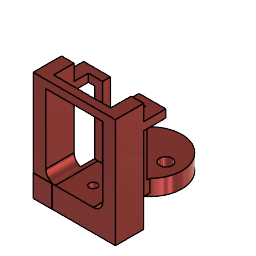
Hexapod Assembly (Autodesk Fusion 360 archive; units mm, degrees)
design "Coxa V1"
part number: 2026-04-28-18-44-43-401
Autodesk Fusion 360 part; units mm, degrees
note: some values were not read from the file. Chosen so that the rebuilt part matches the saved one: which face or edge a step refers to; which pieces of a blend or face edit are solid. Set by a fixed rule: which sketch regions a step uses.
sketch "Sketch1" plane through (0, 0, 0) normal (0, 0, 1) x (1, 0, 0)
sketch "Sketch2" plane through (0, 0, 0) normal (0, 0, 1) x (1, 0, 0)
  circle A0 centre (14.9677, 30.0451) radius 10
  dimension "d1" = 20
  measures "d1" diameter of A0
extrude "Extrude1" add sketch "Sketch2" along normal blind 5
sketch "Sketch3" plane through (0, 0, 5) normal (0, 0, 1) x (-1, 0, 0)
  circle A0 centre (-14.9677, -30.0451) radius 10
  line L0 (-8, -27.0451) -> (-22, -27.0451)
  line L1 (-22, -27.0451) -> (-22, -12.0451)
  line L2 (-22, -12.0451) -> (-8, -12.0451)
  line L3 (-8, -12.0451) -> (-8, -27.0451)
  dimension "d4" = 14
  dimension "d5" = 15
  dimension "d6" = 3
  constraint horizontal L0
  constraint vertical L1
  constraint horizontal L2
  constraint vertical L3
  measures "d4" distance of L0.start L0.end
  measures "d5" distance of L0.start L2.end
  measures "d6" distance of A0.centre L0
extrude "Extrude2" cut sketch "Sketch3" against normal blind 4 contours A0 L0 L1 L3 | A0 L1 L2 L3 picked at (-15.2391, -24.7211)
extrude "Extrude3" add 1 faces at (12.6667, 27.0451, 3.6667) along direction (0, -1, 0) blind 15
sketch "Sketch4" plane through (0, 0, 5) normal (0, 0, 1) x (-1, 0, 0)
extrude "Extrude4" add 1 faces at (12.6667, 12.0451, 3.6667) along direction (0, -1, 0) blind 6
sketch "Sketch5" plane through (8, 0, 0) normal (-1, 0, 0) x (0, -1, 0)
sketch "Sketch6" plane through (0, 0, 5) normal (0, 0, 1) x (1, 0, 0)
sketch "Sketch7" plane through (8, 0, 0) normal (-1, 0, 0) x (0, -1, 0)
sketch "Sketch8" plane through (0, 0, 1) normal (0, 0, -1) x (1, 0, 0)
sketch "Sketch9" plane through (22, 0, 0) normal (1, 0, 0) x (0, 1, 0)
  line L0 (22.9355, 1) -> (22.9355, 5)
  line L1 (22.9355, 5) -> (6.0451, 5)
  line L2 (6.0451, 5) -> (6.0451, 1)
  line L3 (6.0451, 1) -> (22.9355, 1)
  line L4 (15, 1) -> (15, 5)
  constraint coincident L3 L4.start
  constraint coincident L1 L4.end
  constraint perpendicular L1 L4
extrude "Extrude5" add sketch "Sketch9" along normal blind 2.5 contours L1 L2 L3 L4
sketch "Sketch10" plane through (8, 0, 0) normal (-1, 0, 0) x (0, -1, 0)
  line L0 (-15, 1) -> (-6, 1)
  line L1 (-6, 1) -> (-6, 5)
  line L2 (-6, 5) -> (-15, 5)
  line L3 (-15, 5) -> (-15, 1)
  constraint horizontal L0
  constraint vertical L1
  constraint horizontal L2
  constraint vertical L3
extrude "Extrude6" add sketch "Sketch10" along normal blind 2.5
sketch "Sketch11" plane through (8, 0, 0) normal (-1, 0, 0) x (0, -1, 0)
sketch "Sketch12" plane through (0, 0, 5) normal (0, 0, 1) x (-1, 0, 0)
  arc A0 (-22, -22.9355) -> (-8, -22.8721) centre (-14.9677, -30.0451) ccw
  line L0 (-8, -22.8721) -> (-8, -15)
  line L1 (-8, -15) -> (-5.5, -15)
  line L2 (-5.5, -15) -> (-5.5, -6)
  line L3 (-5.5, -6) -> (-8, -6)
  line L4 (-8, -6) -> (-8, -6.0451)
  line L5 (-8, -6.0451) -> (-24.5, -6.0451)
  line L6 (-24.5, -6.0451) -> (-24.5, -15)
  line L7 (-24.5, -15) -> (-22, -15)
  line L8 (-22, -15) -> (-22, -22.9355)
  line L9 (-24.5, -6.0451) -> (-5.5, -6.0451)
  line L10 (-5.5, -6.0451) -> (-5.5, -15)
  line L11 (-5.5, -15) -> (-24.5, -15)
  line L12 (-24.5, -15) -> (-24.5, -6.0451)
  line L13 (-22, -15) -> (-8, -15)
  line L14 (-8, -15) -> (-8, -6)
  line L15 (-8, -6) -> (-22, -6)
  line L16 (-22, -6) -> (-22, -15)
  constraint horizontal L9
  constraint vertical L10
  constraint horizontal L11
  constraint vertical L12
  constraint coincident L1.end L2.start
  constraint coincident L5.end L6.start
  constraint horizontal L13
  constraint vertical L14
  constraint horizontal L15
  constraint vertical L16
  constraint coincident L3.end L4.start
  constraint coincident L7.end L8.start
extrude "Extrude7" add sketch "Sketch12" along normal blind 35 contours L5 L6 L7 L9 L11 L12 L16 | L1 L2 L9 L10 L11 L14
sketch "Sketch13" plane through (0, 0, 40) normal (0, 0, 1) x (-1, 0, 0)
  line L0 (-8, -15) -> (-5.5, -15)
  line L1 (-5.5, -15) -> (-5.5, -6.0451)
  line L2 (-5.5, -6.0451) -> (-8, -6.0451)
  line L3 (-8, -6.0451) -> (-8, -15)
  line L4 (-5.5, -15) -> (-24.5, -15)
  line L5 (-24.5, -15) -> (-24.5, -6)
  line L6 (-24.5, -6) -> (-5.5, -6)
  line L7 (-5.5, -6) -> (-5.5, -15)
  constraint horizontal L4
  constraint vertical L5
  constraint horizontal L6
  constraint vertical L7
  constraint coincident L0.end L1.start
extrude "Extrude8" add sketch "Sketch13" along normal blind 2.5
sketch "Sketch14" plane through (0, 0, 5) normal (0, 0, 1) x (-1, 0, 0)
  circle A0 centre (-10, -30) radius 2
  circle A1 centre (-20, -30) radius 2
  dimension "d21" = 4
  dimension "d22" = 4
  measures "d21" diameter of A0
  measures "d22" diameter of A1
extrude "Extrude9" cut sketch "Sketch14" against normal blind 10
sketch "Sketch15" plane through (0, 0, 5) normal (0, 0, 1) x (-1, 0, 0)
  line L0 (-16.4081, -6.0596) -> (-16.4081, -12.0596)
  line L1 (-24.4681, -12.0596) -> (-5.5251, -12.0596)
  circle A0 centre (-14.9966, -12.0596) radius 1.25
  dimension "d25" = 6
  dimension "d26" = 2.5
  constraint vertical L0
  constraint horizontal L1
  constraint midpoint L1 A0.centre
  measures "d25" distance of L0.start L0.end
  measures "d26" diameter of A0
extrude "Extrude10" cut sketch "Sketch15" against normal blind 10
sketch "Sketch16" plane through (0, 0, 40) normal (0, 0, -1) x (1, 0, 0)
sketch "Sketch17" plane through (0, 0, 42.5) normal (0, 0, 1) x (-1, 0, 0)
  line L0 (-5.5, -6) -> (-24.5, -6)
  line L1 (-24.5, -6) -> (-24.5, -15)
  line L2 (-24.5, -15) -> (-5.5, -15)
  line L3 (-5.5, -15) -> (-5.5, -6)
sketch "Sketch18" plane through (0, 6.0451, 0) normal (0, -1, 0) x (1, 0, 0)
sketch "Sketch19" plane through (0, 0, 1) normal (0, 0, -1) x (1, 0, 0)
sketch "Sketch20" plane through (0, 0, 1) normal (0, 0, -1) x (1, 0, 0)
  circle A0 centre (14.9966, -12.0596) radius 1.25
  arc A1 (22, -22.9355) -> (8, -22.8721) centre (14.9677, -30.0451) ccw
  line L0 (22, -22.9355) -> (22, -15)
  line L1 (22, -15) -> (24.5, -15)
  line L2 (24.5, -15) -> (24.5, -6.0451)
  line L3 (24.5, -6.0451) -> (8, -6.0451)
  line L4 (8, -6.0451) -> (8, -6)
  line L5 (8, -6) -> (5.5, -6)
  line L6 (5.5, -6) -> (5.5, -15)
  line L7 (5.5, -15) -> (8, -15)
  line L8 (8, -15) -> (8, -22.8721)
  line L9 (24.5, -15) -> (5.5, -15)
  line L10 (5.5, -15) -> (5.5, -6)
  line L11 (5.5, -6) -> (24.5, -6)
  line L12 (24.5, -6) -> (24.5, -15)
  constraint horizontal L9
  constraint vertical L10
  constraint horizontal L11
  constraint vertical L12
  constraint coincident L5.end L6.start
  constraint coincident L1.end L2.start
extrude "Extrude11" add sketch "Sketch20" along normal blind 3 contours L1 L2 L3 L4 L5 L6 L7 L9 L10 L11 L12
sketch "Sketch21" plane through (0, 0, 0) normal (0, 0, -1) x (1, 0, 0)
  circle A0 centre (10, -30) radius 2
sketch "Sketch22" plane through (0, 0, 42.5) normal (0, 0, 1) x (-1, 0, 0)
sketch "Sketch23" plane through (0, 0, 0) normal (0, 1, 0) x (1, 0, 0)
sketch "Sketch24" plane through (0, 15, 0) normal (0, 1, 0) x (-1, 0, 0)
sketch "Sketch25" plane through (0, 0, 5) normal (0, 0, 1) x (-1, 0, 0)
sketch "Sketch26" plane through (0, 0, 5) normal (0, 0, 1) x (-1, 0, 0)
  line L0 (-8, -22) -> (-10.5, -22)
  line L1 (-10.5, -22) -> (-10.5, -19.5)
  line L2 (-10.5, -19.5) -> (-8, -19.5)
  line L3 (-8, -19.5) -> (-8, -22)
  line L4 (-22, -22) -> (-19.5, -22)
  line L5 (-19.5, -22) -> (-19.5, -19.5)
  line L6 (-19.5, -19.5) -> (-22, -19.5)
  line L7 (-22, -19.5) -> (-22, -22)
  constraint horizontal L0
  constraint perpendicular L0 L1
  constraint perpendicular L1 L2
  constraint perpendicular L0 L3
  constraint perpendicular L3 L4
  constraint perpendicular L4 L5
  constraint perpendicular L5 L6
  constraint perpendicular L4 L7
sketch "Sketch27" plane through (0, 15, 0) normal (0, 1, 0) x (-1, 0, 0)
extrude "Extrude12" add sketch "Sketch26" along normal blind 22.5
sketch "Sketch28" plane through (22, 0, 0) normal (1, 0, 0) x (0, 1, 0)
  line L0 (15, 5) -> (15, 1)
  line L1 (15, 1) -> (22.9355, 1)
  line L2 (22.9355, 1) -> (22.9355, 5)
  line L3 (22.9355, 5) -> (22, 5)
  line L4 (22, 5) -> (22, 27.5)
  line L5 (22, 27.5) -> (19.5, 27.5)
  line L6 (19.5, 27.5) -> (19.5, 5)
  line L7 (19.5, 5) -> (15, 5)
  line L8 (19.5, 27.5) -> (19.5, 25)
  line L9 (22, 25) -> (19.5, 25)
  line L10 (22, 25) -> (22, 27.5)
  line L11 (22, 27.5) -> (19.5, 27.5)
  constraint coincident L5.end L6.start
  constraint coincident L6 L8.end
  constraint coincident L4 L9.start
  constraint perpendicular L8 L9
  constraint coincident L4.end L5.start
sketch "Sketch29" plane through (22, 0, 0) normal (1, 0, 0) x (0, 1, 0)
sketch "Sketch30" plane through (22, 0, 0) normal (1, 0, 0) x (0, 1, 0)
sketch "Sketch31" plane through (22, 0, 0) normal (1, 0, 0) x (0, 1, 0)
  line L0 (19.5, 25) -> (15, 25)
  line L1 (15, 25) -> (15, 27.5)
  line L2 (15, 27.5) -> (19.5, 27.5)
  line L3 (19.5, 27.5) -> (19.5, 25)
  constraint horizontal L0
  constraint perpendicular L0 L1
  constraint perpendicular L1 L2
  constraint perpendicular L0 L3
extrude "Extrude13" add sketch "Sketch28" sketch "Sketch31" along normal blind 2.5 contours L4 L5 L6 L8 L9 L10 L11 of sketch 2
sketch "Sketch32" plane through (8, 0, 0) normal (-1, 0, 0) x (0, -1, 0)
  line L0 (-15, 1) -> (-15, 5)
  line L1 (-15, 5) -> (-19.5, 5)
  line L2 (-19.5, 5) -> (-19.5, 27.5)
  line L3 (-19.5, 27.5) -> (-22, 27.5)
  line L4 (-22, 27.5) -> (-22, 5)
  line L5 (-22, 5) -> (-22.8721, 5)
  line L6 (-22.8721, 5) -> (-22.8721, 1)
  line L7 (-22.8721, 1) -> (-15, 1)
  line L8 (-15, 25) -> (-22, 25)
  line L9 (-22, 25) -> (-22, 27.5)
  line L10 (-22, 27.5) -> (-15, 27.5)
  constraint coincident L4 L8.end
  constraint perpendicular L4 L8
  constraint coincident L3.end L4.start
  constraint perpendicular L2 L10
sketch "Sketch33" plane through (8, 0, 0) normal (-1, 0, 0) x (0, -1, 0)
sketch "Sketch34" plane through (8, 0, 0) normal (-1, 0, 0) x (0, -1, 0)
  line L0 (-15, 25) -> (-15, 27.5)
  line L1 (-15, 27.5) -> (-19.5, 27.5)
  line L2 (-19.5, 27.5) -> (-19.5, 25)
  line L3 (-19.5, 25) -> (-15, 25)
  constraint vertical L0
  constraint perpendicular L0 L1
  constraint perpendicular L1 L2
  constraint perpendicular L0 L3
extrude "Extrude14" add sketch "Sketch34" sketch "Sketch32" along normal blind 2.5 of sketch 2 contours L2 L3 L4 L8 L9 L10
sketch "Sketch35" plane through (0, 0, 42.5) normal (0, 0, 1) x (-1, 0, 0)
extrude "Extrude15" cut sketch "Sketch17" against normal blind 10
sketch "Sketch36" plane through (0, 0, 32.5) normal (0, 0, 1) x (-1, 0, 0)
  line L0 (-22, -6.0451) -> (-24.5, -6.0451)
  line L1 (-24.5, -6.0451) -> (-24.5, -15)
  line L2 (-24.5, -15) -> (-22, -15)
  line L3 (-22, -15) -> (-22, -6.0451)
  line L4 (-22, -6.0451) -> (-8, -6.0451)
  line L5 (-8, -6.0451) -> (-8, -8.5451)
  line L6 (-8, -8.5451) -> (-22, -8.5451)
  dimension "d39" = 2.5
  constraint coincident L0.start L3.end
  constraint perpendicular L3 L4
  constraint perpendicular L4 L5
  constraint coincident L3 L6.end
  constraint perpendicular L3 L6
  measures "d39" distance of L4.end L5.end
extrude "Extrude16" add sketch "Sketch36" against normal blind 2.5 contours L3 L4 L5 L6
sketch "Sketch37" plane through (0, 0, -2) normal (0, 0, -1) x (1, 0, 0)
  circle A0 centre (14.9966, -12.0596) radius 1.25
  line L0 (24.5, -15) -> (24.5, -6.0451)
  line L1 (24.5, -6.0451) -> (8, -6.0451)
  line L2 (8, -6.0451) -> (8, -6)
  line L3 (8, -6) -> (5.5, -6)
  line L4 (5.5, -6) -> (5.5, -15)
  line L5 (5.5, -15) -> (24.5, -15)
  circle A1 centre (14.9966, -12.0596) radius 1.25
  constraint concentric A0 A1
extrude "Extrude17" add sketch "Sketch37" against normal blind 1 contours A0 A1
extrude "Extrude18" add 1 faces at (5.5, 9.03, 20.8333) along direction (-1, 0, 0) blind 1.5
extrude "Extrude19" add 1 faces at (24.5, 9.03, 18.5) along direction (1, 0, 0) blind 1.5
extrude "Extrude20" cut 1 faces at (22, 9.03, 20) along direction (1, 0, 0) blind 2
extrude "Extrude21" cut 1 faces at (8, 9.03, 20) along direction (-1, 0, 0) blind 2
extrude "Extrude22" add 1 faces at (4, 9.03, 20.8333) along direction (-1, 0, 0) blind 2
extrude "Extrude23" add 1 faces at (26, 9.03, 18.5) along direction (1, 0, 0) blind 2
fillet "Fillet1" radius 3 1 edges at (6, 10.5225, 5)
fillet "Fillet2" radius 3 1 edges at (24, 10.5225, 5)

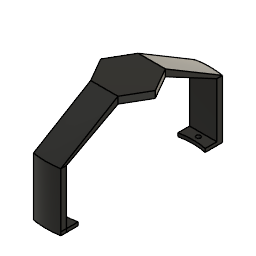
design "cover V2"
part number: 2026-05-21-21-22-30-375
Autodesk Fusion 360 part; units mm, degrees
sketch "Sketch1" plane through (0, 0, 0) normal (0, 0, 1) x (1, 0, 0)
  circle A0 centre (0, 0) radius 60
  dimension "d1" = 120
  constraint coincident A0.centre origin
  measures "d1" diameter of A0
extrude "Extrude1" add sketch "Sketch1" along normal blind 2.5 makes body 1
sketch "Sketch2" plane through (0, 0, 2.5) normal (0, 0, 1) x (-1, 0, 0)
  circle A0 centre (0, 0) radius 60
  line L0 (0, 0) -> (0, -60)
  line L1 (0, 0) -> (0, 60)
  circle A1 centre (0, 0) radius 45
  line L2 (0, -45) -> (-10, -45)
  line L3 (0, -45) -> (10, -45)
  line L4 (10, -45) -> (10, -59.1608)
  line L5 (-10, -45) -> (-10, -59.1608)
  line L6 (0, 45) -> (-10, 45)
  line L7 (0, 45) -> (10, 45)
  line L8 (10, 45) -> (10, 59.1608)
  line L9 (-10, 45) -> (-10, 59.1608)
  line L10 (0, -60) -> (0, -55)
  line L11 (0, -55) -> (-10, -55)
  line L12 (0, -55) -> (10, -55)
  line L13 (0, 60) -> (0, 55)
  line L14 (-10, 55) -> (0, 55)
  line L15 (0, 55) -> (10, 55)
  dimension "d5" = 90
  dimension "d6" = 10
  dimension "d7" = 10
  dimension "d8" = 10
  dimension "d9" = 10
  constraint coincident A0 L0.end
  constraint vertical L0
  constraint coincident A0 L1.end
  constraint parallel L0 L1
  constraint concentric A0 A1
  constraint coincident A1 L2.start
  constraint coincident L0 L2.start
  constraint perpendicular L0 L2
  constraint perpendicular L0 L3
  constraint coincident A0 L4.end
  constraint perpendicular L3 L4
  constraint coincident A0 L5.end
  constraint perpendicular L2 L5
  constraint coincident A1 L6.start
  constraint perpendicular L1 L6
  constraint perpendicular L1 L7
  constraint coincident A0 L8.end
  constraint perpendicular L7 L8
  constraint coincident A0 L9.end
  constraint perpendicular L6 L9
  constraint coincident L0 L10.end
  constraint coincident L5 L11.end
  constraint perpendicular L5 L11
  constraint coincident L4 L12.end
  constraint perpendicular L4 L12
  constraint coincident L1 L13.end
  constraint coincident L9 L14.start
  constraint perpendicular L1 L14
  constraint coincident L8 L15.end
  constraint perpendicular L8 L15
  measures "d5" diameter of A1
  measures "d6" distance of L2.start L2.end
  measures "d7" distance of L2.start L3.end
  measures "d8" distance of L6.start L6.end
  measures "d9" distance of L6.start L7.end
extrude "Extrude2" add sketch "Sketch2" along normal blind 40 contours A0 L1 L8 L13 L15 | A0 L0 L4 L10 L12 | A0 L1 L9 L13 L14 | A0 L0 L5 L10 L11 bodies 1
sketch "Sketch3" plane through (0, 0, 0) normal (1, 0, 0) x (0, 1, 0)
  line L0 (-0.0059, 2.4931) -> (-0.0059, 62.4931)
  line L1 (-0.0059, 62.4931) -> (24.9941, 62.4931)
  line L2 (24.9941, 62.4931) -> (-0.0059, 62.4931)
  line L3 (-0.0059, 62.4931) -> (-25.0059, 62.4931)
  line L4 (-25.0059, 62.4931) -> (-25.0059, 67.4931)
  line L5 (-25.0059, 67.4931) -> (24.9941, 67.4931)
  line L6 (24.9941, 67.4931) -> (24.9941, 62.4931)
  dimension "d12" = 60
  dimension "d13" = 25
  dimension "d14" = 25
  dimension "d15" = 5
  dimension "d16" = 50
  constraint vertical L0
  constraint perpendicular L0 L1
  constraint perpendicular L0 L3
  constraint perpendicular L3 L4
  constraint perpendicular L4 L5
  measures "d12" distance of L0.start L0.end
  measures "d13" distance of L0.end L1.end
  measures "d14" distance of L0.end L3.end
  measures "d15" distance of L3.end L4.end
  measures "d16" distance of L4.end L5.end
extrude "Extrude3" add sketch "Sketch3" along normal blind 20 separate body makes body 2
extrude "Extrude4" add 1 faces at (0, -0.0059, 65.8264) along direction (-1, 0, 0) blind 20 on bodies 2 bodies 2
sketch "Sketch4" plane through (0, 0, 67.4931) normal (0, 0, 1) x (-1, 0, 0)
  line L0 (20, 25.0059) -> (-20, 25.0059)
  line L1 (-20, 25.0059) -> (-20, -24.9941)
  line L2 (-20, -24.9941) -> (20, -24.9941)
  line L3 (20, -24.9941) -> (20, 25.0059)
  line L4 (-9.9944, 17.3237) -> (-20, 0.0064)
  line L5 (-20, 0.0064) -> (-10.0055, -17.3173)
  line L6 (-10.0055, -17.3173) -> (9.9944, -17.3237)
  line L7 (9.9944, -17.3237) -> (20, -0.0064)
  line L8 (20, -0.0064) -> (10.0055, 17.3173)
  line L9 (10.0055, 17.3173) -> (-9.9944, 17.3237)
  dimension "d21" = 20
  measures "d21" distance of L4.start origin
extrude "Extrude5" cut sketch "Sketch4" against normal blind 10 contours L0 L1 L3 L4 L8 L9 | L1 L2 L3 L5 L6 L7 bodies 2
loft "Loft1" add section 1 face at (1.1157, 56.6355, 42.5) section 2 face at (3.3389, 17.3194, 65.8264) on bodies 1 2 bodies 1 2
loft "Loft2" add section 1 face at (-3.3389, -17.3194, 64.1597) section 2 face at (1.1157, -56.6355, 42.5) on bodies 1 bodies 1
sketch "Sketch5" plane through (0, 0, 2.5) normal (0, 0, 1) x (-1, 0, 0)
  line L0 (10, -55) -> (10, -59.1608)
  arc A0 (10, -59.1608) -> (10, 59.1608) centre (0, 0) ccw
  line L1 (10, 59.1608) -> (10, 55)
  line L2 (10, 55) -> (-10, 55)
  line L3 (-10, 55) -> (-10, 59.1608)
  arc A1 (-10, 59.1608) -> (-10, -59.1608) centre (0, 0) ccw
  line L4 (-10, -59.1608) -> (-10, -55)
  line L5 (-10, -55) -> (10, -55)
  circle A2 centre (0, 0) radius 47.5
  line L6 (0, -47.5) -> (0, -51.5)
  line L7 (10, -55) -> (10, -46.4354)
  line L8 (-10, -55) -> (-10, -46.4354)
  line L9 (10, -55) -> (10, -59.1608)
  line L10 (-10, -55) -> (-10, -59.1608)
  line L11 (-10, 55) -> (-10, 46.4354)
  line L12 (10, 55) -> (10, 46.4354)
  line L13 (0, 47.5) -> (0, 51.5)
  circle A3 centre (0, -51.5) radius 1.6
  circle A4 centre (0, 51.5) radius 1.6
  dimension "d24" = 95
  dimension "d27" = 3.2
  dimension "d28" = 3.2
  constraint concentric A0 A2
  constraint coincident A2 L6.start
  constraint perpendicular L5 L6
  constraint coincident L0.start L5.end
  constraint coincident A2 L7.end
  constraint perpendicular L5 L7
  constraint coincident L4.end L5.start
  constraint coincident A2 L8.end
  constraint perpendicular L5 L8
  constraint coincident L0.end A0.start
  constraint coincident A1.end L4.start
  constraint coincident L2.end L3.start
  constraint coincident A2 L11.end
  constraint perpendicular L2 L11
  constraint coincident L1.end L2.start
  constraint coincident A2 L12.end
  constraint perpendicular L2 L12
  constraint coincident A2 L13.start
  constraint perpendicular L2 L13
  constraint coincident L6.end A3.centre
  constraint coincident L13.end A4.centre
  measures "d24" diameter of A2
  measures "d27" diameter of A3
  measures "d28" diameter of A4
extrude "Extrude6" cut sketch "Sketch5" against normal blind 10 contours L0 A0 L1 A2 L7 L9 L12 | L3 A1 L4 A2 L8 L10 L11 | A2 | A3 | A4 bodies 1
